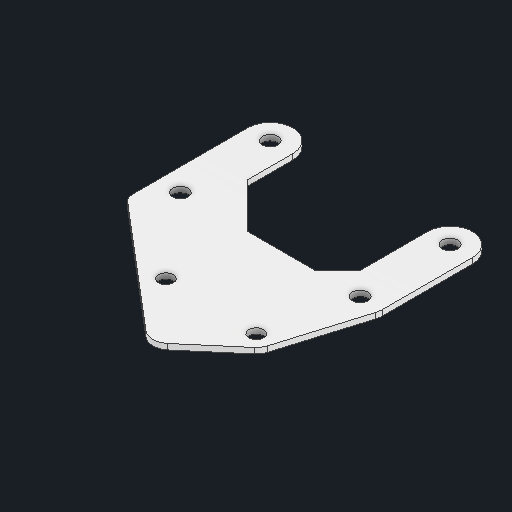
# Autodesk Inventor part: gusset
Saved by Autodesk Inventor 2025 (Build 290162000, 162)
## iProperties
Created: 2024-10-04
Part Number: gusset
Material: Acetal Resin, White
Document SubType Name: Modeling
Designer: Averey Ku
Density: 1.425 g/cm^3
Appearance: Smooth - White
Author: Averey Ku
Autodesk Inventor part; units mm, degrees
ref_plane "YZ Plane" through (0, 0, 0) normal (1, 0, 0) x (0, 1, 0)
ref_plane "XZ Plane" through (0, 0, 0) normal (0, 1, 0) x (-1, 0, 0)
ref_plane "XY Plane" through (0, 0, 0) normal (0, 0, 1) x (1, 0, 0)
sketch "main" plane through (0, 0, 0) normal (0, 0, 1) x (1, 0, 0)
  circle A0 centre (9.0037, 34.4943) radius 2.1844
  line L0 (21.7037, 28.1443) -> (9.0037, 15.4443)
  line L1 (34.4037, 28.1443) -> (21.7037, 28.1443)
  line L2 (1.7426, 40.8443) -> (9.0037, 40.8443)
  line L3 (9.0037, 40.8443) -> (34.4037, 40.8443)
  circle A1 centre (34.4037, 34.4943) radius 2.1844
  arc A2 (34.4037, 28.1443) -> (34.4037, 40.8443) centre (34.4037, 34.4943) ccw
  arc A3 (-18.4336, -13.8478) -> (-16.1882, -15.3171) centre (-14.8088, -10.7587) ccw
  circle A4 centre (-14.8088, -10.7587) radius 2.0828
  line L4 (-16.1882, -15.3171) -> (7.1645, -22.3836)
  circle A5 centre (-14.1255, 15.4716) radius 2.0828
  line L5 (-29.6834, -0.6474) -> (-18.4336, -13.8478)
  arc A6 (-29.6904, 5.5225) -> (-29.6834, -0.6474) centre (-26.0586, 2.4417) ccw
  line L6 (-0.6786, 39.7231) -> (-29.6904, 5.5225)
  line L7 (9.0037, -3.6057) -> (9.0037, 15.4443)
  line L8 (15.3537, -9.9557) -> (34.4037, -9.9557)
  line L9 (15.3537, -9.9557) -> (9.0037, -3.6057)
  circle A7 centre (34.4037, -16.3057) radius 2.1844
  arc A8 (34.4037, -22.6557) -> (34.4037, -9.9557) centre (34.4037, -16.3057) ccw
  circle A9 centre (9.0037, -16.3057) radius 2.1844
  arc A10 (7.1645, -22.3836) -> (9.0037, -22.6557) centre (9.0037, -16.3057) ccw
  line L10 (9.0037, -22.6557) -> (34.4037, -22.6557)
  arc A11 (1.7426, 40.8443) -> (-0.6786, 39.7231) centre (1.7426, 37.6693) ccw
  point P0 (6.3419, 6.6617)
  point P1 (9.0037, 28.1443)
  point P2 (0.2724, 40.8443)
  point P3 (-32.3099, 2.4346)
  point P4 (9.0037, -9.9557)
  dimension "d0" = 4.1656
  dimension "d1" = 9.525
  dimension "d2" = 12.7
  dimension "d3" = 12.7
  dimension "d4" = 6.35
  dimension "d5" = 6.35
  dimension "d6" = 4.1656
  dimension "d7" = 4.7625
  dimension "d8" = 8.7312
  dimension "d9" = 3.175
  dimension "d12" = 49.2125
  measures "d0" diameter of A4
  measures "d1" diameter of A3
  measures "d2" distance of L1.end point (9.004, 28.144)
  measures "d3" distance of L7.end point (9.004, 28.144)
  measures "d4" distance of L8.start point (9.004, -9.956)
  measures "d5" distance of L7.start point (9.004, -9.956)
  measures "d6" diameter of A5
  measures "d7" radius of A6
  measures "d8" distance of point (0.272, 40.844) L2.end
  measures "d9" radius of A11
  measures "d12" horizontal distance of A3.centre A2.centre
sketch "Sketch1" plane through (0, 0, 0) normal (0, 1, 0) x (-1, 0, 0)
  circle A0 centre (0.0003, 25.4) radius 2.1844
  line L0 (-6.3499, 12.7001) -> (-19.0497, 25.4002)
  line L1 (-6.35, 0.0001) -> (-6.3499, 12.7001)
  line L2 (6.3503, 32.661) -> (6.3503, 25.3999)
  line L3 (6.3503, 25.3999) -> (6.35, -0.0001)
  circle A1 centre (0, 0) radius 2.1844
  arc A2 (-6.35, 0.0001) -> (6.35, -0.0001) centre (0, 0) ccw
  arc A3 (-48.3415, 52.8378) -> (-49.8108, 50.5924) centre (-45.2525, 49.213) ccw
  circle A4 centre (-45.2525, 49.213) radius 2.0828
  line L4 (-49.8108, 50.5924) -> (-56.8775, 27.2397)
  circle A5 centre (-19.0222, 48.5293) radius 2.0828
  line L5 (-35.141, 64.0874) -> (-48.3415, 52.8378)
  arc A6 (-28.9711, 64.0944) -> (-35.141, 64.0874) centre (-32.0519, 60.4626) ccw
  line L6 (5.2292, 35.0822) -> (-28.9711, 64.0944)
  line L7 (-38.0997, 25.4004) -> (-19.0497, 25.4002)
  line L8 (-44.4498, 19.0505) -> (-44.45, 0.0005)
  line L9 (-44.4498, 19.0505) -> (-38.0997, 25.4004)
  circle A7 centre (-50.8, 0.0005) radius 2.1844
  arc A8 (-57.15, 0.0006) -> (-44.45, 0.0005) centre (-50.8, 0.0005) ccw
  circle A9 centre (-50.7997, 25.4005) radius 2.1844
  arc A10 (-56.8775, 27.2397) -> (-57.1497, 25.4006) centre (-50.7997, 25.4005) ccw
  line L10 (-57.1497, 25.4006) -> (-57.15, 0.0006)
  arc A11 (6.3503, 32.661) -> (5.2292, 35.0822) centre (3.1753, 32.661) ccw
  point P0 (0, 0)
  point P1 (6.3503, 25.3999)
  constraints: 1 other
extrude "Extrusion1" add sketch "Sketch1" along normal blind 1.5875
equation "\"d3\" = d2"
equation "\"d5\" = d4"
body "Solid1"
